Push_button_PTS820 J20KP SMTR LFS v1 (Autodesk Fusion 360 design; units mm, degrees)
Autodesk Fusion 360 part; units mm, degrees
sketch "Sketch1" plane through (0, 0, 0) normal (0, 0, 1) x (1, 0, 0)
  line L0 (1.45, 1.95) -> (-1.45, 1.95)
  line L1 (-1.45, 1.95) -> (-1.45, -1.95)
  line L2 (-1.45, -1.95) -> (1.45, -1.95)
  line L3 (1.45, -1.95) -> (1.45, 1.95)
  line L4 (1.45, 1.95) -> (-1.45, -1.95) construction
  line L5 (-1.45, 1.95) -> (1.45, -1.95) construction
  dimension "d1" = 2.9
  dimension "d2" = 3.9
  constraint horizontal L0
  constraint perpendicular L0 L1
  constraint parallel L0 L2
  constraint parallel L1 L3
  constraint coincident L4 origin
  constraint coincident L5 origin
  measures "d1" distance of L1.end L2.end
  measures "d2" distance of L0.end L1.end
extrude "Extrude1" add sketch "Sketch1" along normal blind 1.5 makes body 1
fillet "Fillet1" radius 0.3 8 edges at (0, 1.95, 1.5) (0, -1.95, 1.5) (1.45, 0, 1.5) (-1.45, 0, 1.5) (1.45, -1.95, 0.75) (-1.45, -1.95, 0.75) (1.45, 1.95, 0.75) (-1.45, 1.95, 0.75) on bodies 1
sketch "Sketch2" plane through (0, 0, 1.5) normal (0, 0, 1) x (-1, 0, 0)
  line L0 (1.15, -1.65) -> (1.15, 1.65)
  line L1 (1.15, 1.65) -> (-1.15, 1.65)
  line L2 (-1.15, 1.65) -> (-1.15, -1.65)
  line L3 (-1.15, -1.65) -> (1.15, -1.65)
  circle A0 centre (0, 0) radius 1
  dimension "d7" = 2
  constraint coincident A0.centre origin
  measures "d7" diameter of A0
extrude "Extrude2" add sketch "Sketch2" along normal blind 1 separate body contours A0 makes body 2
fillet "Fillet2" radius 0.1 1 edges at (0.9323, 0.3616, 2.5) on bodies 2
